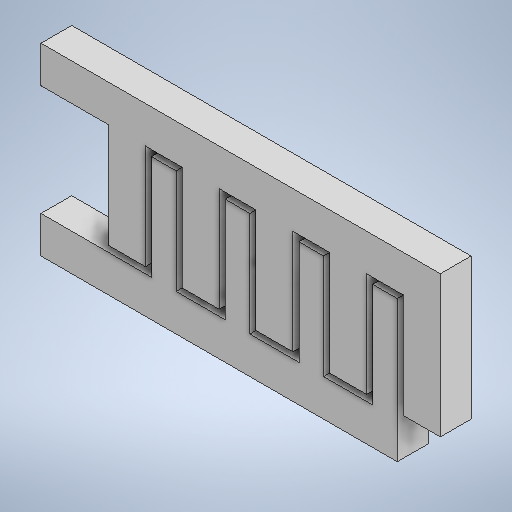
# Autodesk Inventor part: Sensor
Saved by Autodesk Inventor 2025.2 (Build 292293000, 293)
## iProperties
Created: 2025-03-19
Part Number: Sensor
Material: Generic
Document SubType Name: Modeling
Designer: ishad
Density: 1 g/cm^3
Appearance: Default
Author: ishad
Autodesk Inventor part; units mm, degrees
ref_plane "YZ Plane" through (0, 0, 0) normal (1, 0, 0) x (0, 1, 0)
ref_plane "XZ Plane" through (0, 0, 0) normal (0, 1, 0) x (-1, 0, 0)
ref_plane "XY Plane" through (0, 0, 0) normal (0, 0, 1) x (1, 0, 0)
sketch "Sketch1" plane through (0, 0, 0) normal (0, 0, 1) x (1, 0, 0)
  line L0 (-6.5647, 31.3909) -> (-6.5647, 8.3909)
  line L1 (-6.5647, 8.3909) -> (-12.5647, 8.3909)
  line L2 (-18.5647, 8.3909) -> (-24.5647, 8.3909)
  line L3 (-30.5647, 8.3909) -> (-36.5647, 8.3909)
  line L4 (-54.5647, 8.3909) -> (-60.5647, 8.3909)
  line L5 (-6.5647, 31.3909) -> (-71.5647, 31.3909)
  line L6 (-71.5647, 31.3909) -> (-71.5647, 25.3909)
  line L7 (-71.5647, 25.3909) -> (-60.5647, 25.3909)
  line L8 (-60.5647, 25.3909) -> (-60.5647, 8.3909)
  line L9 (-54.5647, 8.3909) -> (-54.5647, 25.3909)
  line L10 (-54.5647, 25.3909) -> (-48.5647, 25.3909)
  line L11 (-48.5647, 25.3909) -> (-48.5647, 8.3909)
  line L12 (-48.5647, 8.3909) -> (-42.5647, 8.3909)
  line L13 (-42.5647, 8.3909) -> (-42.5647, 25.3909)
  line L14 (-42.5647, 25.3909) -> (-36.5647, 25.3909)
  line L15 (-36.5647, 25.3909) -> (-36.5647, 8.3909)
  line L16 (-30.5647, 8.3909) -> (-30.5647, 25.3909)
  line L17 (-30.5647, 25.3909) -> (-24.5647, 25.3909)
  line L18 (-24.5647, 25.3909) -> (-24.5647, 8.3909)
  line L19 (-18.5647, 8.3909) -> (-18.5647, 25.3909)
  line L20 (-18.5647, 25.3909) -> (-12.5647, 25.3909)
  line L21 (-12.5647, 25.3909) -> (-12.5647, 8.3909)
  line L22 (-71.5647, 7.3909) -> (-71.5647, 1.3909)
  line L23 (-53.5647, 7.3909) -> (-53.5647, 24.3909)
  line L24 (-53.5647, 24.3909) -> (-49.5647, 24.3909)
  line L25 (-49.5647, 24.3909) -> (-49.5647, 7.3909)
  line L26 (-49.5647, 7.3909) -> (-49.5647, 7.3909)
  line L27 (-49.5647, 7.3909) -> (-41.5647, 7.3909)
  line L28 (-41.5647, 24.3909) -> (-37.5647, 24.3909)
  line L29 (-37.5647, 24.3909) -> (-37.5647, 7.3909)
  line L30 (-13.5647, 1.3909) -> (-13.5647, 24.3909)
  line L31 (-13.5647, 24.3909) -> (-17.5647, 24.3909)
  line L32 (-17.5647, 24.3909) -> (-17.5647, 7.3909)
  line L33 (-17.5647, 7.3909) -> (-25.5647, 7.3909)
  line L34 (-25.5647, 7.3909) -> (-25.5647, 24.3909)
  line L35 (-25.5647, 24.3909) -> (-29.5647, 24.3909)
  line L36 (-29.5647, 24.3909) -> (-29.5647, 7.3909)
  line L37 (-29.5647, 7.3909) -> (-37.5647, 7.3909)
  line L38 (-71.5647, 1.3909) -> (-13.5647, 1.3909)
  line L39 (-41.5647, 24.3909) -> (-41.5647, 7.3909)
  line L40 (-71.5647, 7.3909) -> (-53.5647, 7.3909)
  point P0 (0, 0)
  point P1 (-39.0647, 31.3909)
  point P2 (-15.5647, 24.3909)
  dimension "d119" = 6
  dimension "d120" = 6
  dimension "d121" = 17
  dimension "d122" = 23
  dimension "d124" = 65
  dimension "d127" = 31.3909
  dimension "d128" = 71.5648
  dimension "d129" = 6
  dimension "d131" = 6
  dimension "d132" = 1
  constraints: 82 end point, 17 perpendicular, 9 equal length, 9 horizontal, 9 vertical, 7 point on line, 2 midpoint, 1 collinear
  measures "d119" distance of L5.end L6.end
  measures "d120" distance of L22.start L22.end
  measures "d121" distance of L7.end L4.end
  measures "d122" distance of L0.start L0.end
  measures "d124" distance of L0.start L5.end
  measures "d127" distance from line of point (0, 0) L5
  measures "d128" distance from line of point (0, 0) L6
  measures "d129" distance between parallel lines of L0 L21
  measures "d131" distance between parallel lines of L5 L20
  measures "d132" distance from line of L20 point (-15.565, 24.391)
extrude "Extrusion1" add sketch "Sketch1" along normal blind 5
body "Solid1"
